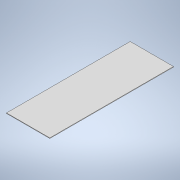
# Autodesk Inventor part: coil_layer_base
Saved by Autodesk Inventor 2020 (Build 240168000, 168)
## iProperties
Created: 2021-01-27
Part Number: coil_layer_base
Material: Generic
Document SubType Name: Modeling
Designer: abij996
Density: 1 g/cm^3
Appearance: Default
Author: abij996
Autodesk Inventor part; units mm, degrees
ref_plane "YZ Plane" through (0, 0, 0) normal (1, 0, 0) x (0, 1, 0)
ref_plane "XZ Plane" through (0, 0, 0) normal (0, 1, 0) x (-1, 0, 0)
ref_plane "XY Plane" through (0, 0, 0) normal (0, 0, 1) x (1, 0, 0)
sketch "Sketch1" plane through (0, 0, 0) normal (0, 1, 0) x (-1, 0, 0)
  line L0 (62.6562, 145.0315) -> (-287.3438, 145.0315)
  line L1 (-287.3438, 145.0315) -> (-287.3438, -854.9685)
  line L2 (-287.3438, -854.9685) -> (62.6562, -854.9685)
  line L3 (62.6562, -854.9685) -> (62.6562, 145.0315)
  point P0 (0, 0)
  dimension "d0" = 1000
  dimension "d1" = 350
  constraints: 8 end point, 2 parallel, 1 horizontal, 1 perpendicular
  measures "d0" distance of L2.end L0.start
  measures "d1" distance of L0.start L0.end
extrude "Extrusion1" add sketch "Sketch1" along normal blind 4.5
body "Solid1"
